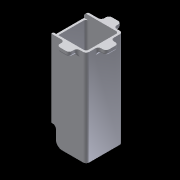
# Autodesk Inventor part: Part3
Saved by Autodesk Inventor 2012 (Build 160160000, 160)
## iProperties
Created: 2012-10-11
Part Number: Part3
Material: Default
Document SubType Name: Modeling
Designer: SONY
Density: 1 g/cm^3
Author: SONY
Autodesk Inventor part; units mm, degrees
ref_plane "YZ Plane" through (0, 0, 0) normal (1, 0, 0) x (0, 1, 0)
ref_plane "XZ Plane" through (0, 0, 0) normal (0, 1, 0) x (-1, 0, 0)
ref_plane "XY Plane" through (0, 0, 0) normal (0, 0, 1) x (1, 0, 0)
sketch "Sketch1" plane through (0, 0, 0) normal (0, 0, 1) x (1, 0, 0)
  line L0 (-50.8, 30.4821) -> (-50.8, -23.4929) projected
  arc A0 (-50.8, -23.4929) -> (-47.625, -26.6679) centre (-47.625, -23.4929) ccw projected
  line L1 (-47.625, -26.6679) -> (47.625, -26.6679) projected
  arc A1 (47.625, -26.6679) -> (50.8, -23.4929) centre (47.625, -23.4929) ccw projected
  line L2 (50.8, -23.4929) -> (50.8, 30.4821) projected
  line L3 (50.8, 30.4821) -> (25.4, 30.4821) projected
  line L4 (25.4, 30.4821) -> (25.4, 1.9071) projected
  arc A2 (22.225, -1.2679) -> (25.4, 1.9071) centre (22.225, 1.9071) ccw projected
  line L5 (22.225, -1.2679) -> (-22.225, -1.2679) projected
  arc A3 (-25.4, 1.9071) -> (-22.225, -1.2679) centre (-22.225, 1.9071) ccw projected
  line L6 (-25.4, 1.9071) -> (-25.4, 30.4821) projected
  line L7 (-25.4, 30.4821) -> (-50.8, 30.4821) projected
  arc A4 (-47.625, 87.6321) -> (-50.8, 84.4571) centre (-47.625, 84.4571) ccw projected
  line L8 (-50.8, 30.4821) -> (-50.8, 84.4571) projected
  line L9 (-25.4, 30.4821) -> (-50.8, 30.4821) projected
  line L10 (-25.4, 59.0571) -> (-25.4, 30.4821) projected
  arc A5 (-22.225, 62.2321) -> (-25.4, 59.0571) centre (-22.225, 59.0571) ccw projected
  line L11 (22.225, 62.2321) -> (-22.225, 62.2321) projected
  arc A6 (25.4, 59.0571) -> (22.225, 62.2321) centre (22.225, 59.0571) ccw projected
  line L12 (25.4, 30.4821) -> (25.4, 59.0571) projected
  line L13 (50.8, 30.4821) -> (25.4, 30.4821) projected
  line L14 (50.8, 84.4571) -> (50.8, 30.4821) projected
  arc A7 (50.8, 84.4571) -> (47.625, 87.6321) centre (47.625, 84.4571) ccw projected
  line L15 (-47.625, 87.6321) -> (47.625, 87.6321) projected
  line L16 (51.435, 0.6371) -> (24.765, 0.6371)
  line L17 (24.765, 0.6371) -> (24.765, 60.3271)
  line L18 (24.765, 60.3271) -> (51.435, 60.3271)
  line L19 (51.435, 60.3271) -> (51.435, 0.6371)
  line L20 (53.185, 0.6371) -> (23.015, 0.6371)
  line L21 (23.015, 0.6371) -> (23.015, 60.3271)
  line L22 (23.015, 60.3271) -> (53.185, 60.3271)
  line L23 (53.185, 60.3271) -> (53.185, 0.6371)
  point P0 (0, 0)
  dimension "d0" = 59.69
  dimension "d1" = 1.905
  dimension "d2" = 26.67
  dimension "d3" = 0.635
  dimension "d4" = 1.75
  dimension "d5" = 1.75
  constraints: 16 end point, 4 parallel, 2 collinear, 2 horizontal, 2 perpendicular
  measures "d0" distance of L18.end L16.start
  measures "d1" distance between parallel lines of L5 L16
  measures "d2" distance between parallel lines of L17 L19
  measures "d3" distance between parallel lines of L4 L17
  measures "d4" distance between parallel lines of L17 L21
  measures "d5" distance between parallel lines of L19 L23
extrude "Extrusion1" add sketch "Sketch1" against normal blind 26.035 contours L19 L22 L23 L20 | L20 L21 L22 L17
sketch "Sketch2" plane through (0, 0, 0) normal (0, 0, 1) x (1, 0, 0)
  line L0 (51.435, 60.3271) -> (51.435, 0.6371) projected
  line L1 (53.185, 0.6371) -> (51.435, 0.6371) projected
  line L2 (53.185, 60.3271) -> (53.185, 0.6371) projected
  line L3 (51.435, 60.3271) -> (53.185, 60.3271) projected
  line L4 (24.765, 0.6371) -> (24.765, 60.3271) projected
  line L5 (23.015, 60.3271) -> (24.765, 60.3271) projected
  line L6 (23.015, 0.6371) -> (23.015, 60.3271) projected
  line L7 (24.765, 0.6371) -> (23.015, 0.6371) projected
  point P0 (0, 0)
extrude "Extrusion2" add sketch "Sketch2" along normal blind 0.635
sketch "Sketch3" plane through (0, 0, 0.635) normal (0, 0, 1) x (1, 0, 0)
  line L0 (24.765, 0.6371) -> (23.015, 0.6371) projected
  line L1 (24.765, 60.3271) -> (24.765, 0.6371) projected
  line L2 (23.015, 60.3271) -> (24.765, 60.3271) projected
  line L3 (23.015, 0.6371) -> (23.015, 60.3271) projected
  line L4 (23.015, 60.3271) -> (53.185, 60.3271)
  line L5 (53.185, 60.3271) -> (53.185, 0.6371)
  line L6 (53.185, 0.6371) -> (23.015, 0.6371)
  line L7 (23.015, 0.6371) -> (23.015, 60.3271)
  point P0 (0, 0)
  constraints: 8 end point, 2 parallel, 1 horizontal, 1 perpendicular
extrude "Extrusion3" add sketch "Sketch3" along normal blind 1.75
sketch "Sketch4" plane through (0, 0, -26.035) normal (0, 0, -1) x (-1, 0, 0)
  line L0 (-51.435, 0.6371) -> (-51.435, 60.3271) projected
  line L1 (-53.185, 60.3271) -> (-51.435, 60.3271) projected
  line L2 (-53.185, 0.6371) -> (-53.185, 60.3271) projected
  line L3 (-51.435, 0.6371) -> (-53.185, 0.6371) projected
  line L4 (-53.185, 60.3271) -> (-23.015, 60.3271)
  line L5 (-23.015, 60.3271) -> (-23.015, 0.6371)
  line L6 (-23.015, 0.6371) -> (-53.185, 0.6371)
  line L7 (-53.185, 0.6371) -> (-53.185, 60.3271)
  point P0 (0, 0)
  constraints: 8 end point, 2 parallel, 1 horizontal, 1 perpendicular
extrude "Extrusion4" add sketch "Sketch4" along normal blind 1.75
sketch "Sketch5" plane through (0, 0, -27.785) normal (0, 0, -1) x (-1, 0, 0)
  line L0 (-53.185, 60.3271) -> (-23.015, 60.3271) projected
  line L1 (-28.3525, 60.3271) -> (-28.3525, 60.3271)
  line L2 (-23.015, 60.3271) -> (-23.015, 0.6371) projected
  line L3 (-53.185, 60.3271) -> (-23.015, 60.3271)
  line L4 (-23.015, 60.3271) -> (-23.015, 64.1371)
  line L5 (-23.015, 64.1371) -> (-53.185, 64.1371)
  line L6 (-53.185, 64.1371) -> (-53.185, 60.3271)
  point P0 (0, 0)
  dimension "d45" = 3.81
  constraints: 10 end point, 2 parallel, 2 perpendicular, 1 collinear, 1 horizontal, 1 point on line
  measures "d45" distance between parallel lines of L3 L5
extrude "Extrusion5" add sketch "Sketch5" against normal blind 1.75
sketch "Sketch6" plane through (0, 0, 2.385) normal (0, 0, 1) x (1, 0, 0)
  line L0 (51.435, 0.6371) -> (51.435, 60.3271) projected
  line L1 (53.185, 60.3271) -> (51.435, 60.3271) projected
  line L2 (24.765, 60.3271) -> (24.765, 0.6371) projected
  line L3 (51.435, 0.6371) -> (24.765, 0.6371) projected
  line L4 (53.185, 60.3271) -> (27.785, 60.3271)
  line L5 (53.185, 64.1371) -> (53.185, 60.3271) projected
  line L6 (23.015, 64.1371) -> (53.185, 64.1371) projected
  line L7 (23.015, 60.3271) -> (23.015, 64.1371) projected
  line L8 (24.765, 60.3271) -> (23.015, 60.3271) projected
  point P0 (0, 0)
  constraints: 2 end point, 1 parallel
extrude "Extrusion6" add sketch "Sketch6" against normal blind 1.75
sketch "Sketch7" plane through (53.185, 0.6371, 2.385) normal (1, 0, 0) x (0, 0, -1)
  line L0 (1.75, 63.5) -> (1.75, 59.69)
  line L1 (28.42, 59.69) -> (1.75, 59.69)
  line L2 (1.75, 59.69) -> (1.75, 63.5)
  line L3 (1.75, 63.5) -> (28.42, 63.5)
  line L4 (28.42, 63.5) -> (28.42, 59.69)
  point P0 (2.385, -0.6371)
  constraints: 10 end point, 2 parallel, 1 horizontal, 1 perpendicular
extrude "Extrusion7" add sketch "Sketch7" against normal blind 1.75
sketch "Sketch8" plane through (0, 0, -27.785) normal (0, 0, -1) x (-1, 0, 0)
  line L0 (-53.185, 0.6371) -> (-28.3525, 0.6371)
  line L1 (-28.3525, 0.6371) -> (-28.3525, -9.5229)
  line L2 (-33.4325, -14.6029) -> (-53.185, -14.6029)
  line L3 (-53.185, -14.6029) -> (-53.185, 0.6371)
  arc A0 (-33.4325, -14.6029) -> (-28.3525, -9.5229) centre (-33.4325, -9.5229) ccw
  line L4 (-23.015, 64.1371) -> (-23.015, 0.6371) projected
  point P0 (0, 0)
  dimension "d26" = 15.24
  dimension "d29" = 5.08
  dimension "d56" = 5.3375
  constraints: 8 end point, 2 parallel, 2 point on circle, 2 tangent, 1 centre point, 1 horizontal, 1 perpendicular
  measures "d26" distance between parallel lines of L0 L2
  measures "d29" radius of A0
  measures "d56" distance between parallel lines of L4 L1
extrude "Lip-1" add sketch "Sketch8" against normal blind 1.75
sketch "Sketch9" plane through (0, 0, 2.385) normal (0, 0, 1) x (1, 0, 0)
  line L0 (51.435, 0.6371) -> (51.435, 64.1371) projected
  line L1 (24.765, 60.3271) -> (24.765, 0.6371) projected
  line L2 (28.3525, 0.6371) -> (24.765, 0.6371) projected
  line L3 (28.3525, -9.5229) -> (28.3525, 0.6371) projected
  arc A0 (28.3525, -9.5229) -> (33.4325, -14.6029) centre (33.4325, -9.5229) ccw projected
  line L4 (53.185, -14.6029) -> (33.4325, -14.6029) projected
  line L5 (53.185, 0.6371) -> (53.185, -14.6029) projected
  line L6 (51.435, 0.6371) -> (53.185, 0.6371) projected
  line L7 (53.185, 0.6371) -> (28.3525, 0.6371)
  line L8 (23.015, 64.1371) -> (51.435, 64.1371) projected
  line L9 (23.015, 60.3271) -> (23.015, 64.1371) projected
  line L10 (24.765, 60.3271) -> (23.015, 60.3271) projected
  point P0 (0, 0)
  constraints: 2 end point, 1 collinear
extrude "Lip-2" add sketch "Sketch9" against normal blind 1.75 contours L6 L5 L4 A0 L3 L7
sketch "Sketch10" plane through (53.185, 0.6371, 0.635) normal (1, 0, 0) x (0, 0, -1)
  line L0 (0, 0) -> (26.67, 0)
  line L1 (26.67, 0) -> (26.67, -15.24)
  line L2 (26.67, -15.24) -> (0, -15.24)
  line L3 (0, -15.24) -> (0, 0)
  point P0 (0.635, -0.6371)
  constraints: 8 end point, 2 parallel, 1 horizontal, 1 perpendicular
extrude "Extrusion10" add sketch "Sketch10" against normal blind 1.75
fillet "Fillet1" radius 2.5 6 edges at (53.185, 24.7671, 2.385) (53.185, 24.7671, -27.785) (23.015, 64.1371, 1.51) (23.015, 64.1371, -26.91) (23.015, 32.3871, 2.385) (23.015, 32.3871, -27.785)
fillet "Fillet1" radius 2 4 edges at (51.435, 24.7671, -26.035) (51.435, 24.7671, 0.635) (24.765, 30.4821, -26.035) (24.765, 30.4821, 0.635)
sketch "Sketch11" plane through (0, 0, 2.385) normal (0, 0, 1) x (1, 0, 0)
  line L0 (53.185, -14.6029) -> (53.185, 64.1371) projected
  line L1 (35.405, 64.1371) -> (45.565, 64.1371)
  line L2 (45.565, 64.1371) -> (45.565, 60.3271)
  line L3 (45.565, 60.3271) -> (35.405, 60.3271)
  line L4 (35.405, 60.3271) -> (35.405, 64.1371)
  line L5 (50.685, 64.1371) -> (25.515, 64.1371) projected
  line L6 (19.215, 60.3271) -> (56.985, 60.3271) projected
  point P0 (0, 0)
  dimension "d36" = 10.16
  dimension "d37" = 7.62
  constraints: 8 end point, 2 collinear, 2 parallel, 1 horizontal, 1 perpendicular
  measures "d36" distance of L1.start L1.end
  measures "d37" distance between parallel lines of L0 L2
extrude "Nub1" add sketch "Sketch11" along normal blind 6.35
sketch "Sketch12" plane through (0, 0, -27.785) normal (0, 0, -1) x (-1, 0, 0)
  line L0 (-35.405, 64.1371) -> (-45.565, 64.1371) projected
  line L1 (-45.565, 60.3271) -> (-35.405, 60.3271) projected
  line L2 (-45.565, 64.1371) -> (-45.565, 60.3271) projected
  line L3 (-35.405, 60.3271) -> (-35.405, 64.1371) projected
  point P0 (0, 0)
  dimension "d47" = 10.16
  measures "d47" distance of L1.start L1.end
extrude "Nub2" add sketch "Sketch12" along normal blind 6.35
sketch "Sketch13" plane through (53.185, -14.6029, -25.285) normal (1, 0, 0) x (0, 0, -1)
  line L0 (0, 78.74) -> (-25.17, 78.74) projected
  line L1 (-25.17, 0) -> (0, 0) projected
  line L2 (-12.585, 78.74) -> (-12.585, 62.2574) construction
  line L3 (-17.665, 78.74) -> (-7.505, 78.74) construction
  line L4 (-7.505, 78.74) -> (-7.505, 74.93) construction
  line L5 (-7.505, 74.93) -> (-17.665, 74.93) construction
  line L6 (-17.665, 74.93) -> (-17.665, 78.74) construction
  line L7 (-39.1575, 72.93) -> (-39.1575, 74.93) construction
  line L8 (-39.1575, 72.93) -> (13.9875, 72.93) construction
  line L9 (13.9875, 74.93) -> (13.9875, 72.93) construction
  line L10 (-39.1575, 74.93) -> (13.9875, 74.93) construction
  line L11 (-17.665, 74.93) -> (-7.505, 74.93)
  line L12 (-7.505, 74.93) -> (-7.505, 78.74)
  line L13 (-7.505, 78.74) -> (-17.665, 78.74)
  line L14 (-17.665, 78.74) -> (-17.665, 74.93)
  point P0 (-25.285, 14.6029)
  dimension "d48" = 10.16
  dimension "d49" = 5.08
  constraints: 18 end point, 4 parallel, 3 perpendicular, 2 horizontal, 1 collinear, 1 midpoint, 1 point on line
  measures "d48" distance between parallel lines of L4 L6
  measures "d49" distance between parallel lines of L2 L6
extrude "Nub-3" add sketch "Sketch13" along normal blind 6.35
fillet "Nub-fillet" radius 2.5 12 edges at (59.535, 62.2321, -7.62) (59.535, 62.2321, -17.78) (53.185, 62.2321, -17.78) (53.185, 62.2321, -7.62) (45.565, 62.2321, 2.385) (45.565, 62.2321, 8.735) (35.405, 62.2321, 8.735) (35.405, 62.2321, 2.385) (35.405, 62.2321, -27.785) (45.565, 62.2321, -27.785) (35.405, 62.2321, -34.135) (45.565, 62.2321, -34.135)
fillet "Nub-fillet" radius 1.25 3 edges at (40.485, 60.3271, -27.785) (53.185, 60.3271, -12.7) (40.485, 60.3271, 2.385)
fillet "Nub-fllet2" radius 1.5 27 edges at (44.8328, 60.3271, -33.4028) (45.565, 60.3271, -30.96) (45.6502, 60.3271, -29.638) (46.9141, 59.8663, -28.0657) (36.1372, 60.3271, -33.4028) (35.405, 60.3271, -30.96) (35.3198, 60.3271, -29.638) (34.0559, 59.8663, -28.0657) (40.485, 60.3271, -34.135) (56.36, 60.3271, -17.78) (55.038, 60.3271, -17.8652) (53.4657, 59.8663, -19.1291) (59.535, 60.3271, -12.7) (58.8028, 60.3271, -8.3522) (56.36, 60.3271, -7.62) (55.038, 60.3271, -7.5348) (53.4657, 59.8663, -6.2709) (58.8028, 60.3271, -17.0478) (36.1372, 60.3271, 8.0028) (35.405, 60.3271, 5.56) (35.3198, 60.3271, 4.238) (34.0559, 59.8663, 2.6657) (44.8328, 60.3271, 8.0028) (45.565, 60.3271, 5.56) (45.6502, 60.3271, 4.238) (46.9141, 59.8663, 2.6657) (40.485, 60.3271, 8.735)
fillet "lip-fillet" radius 2.5 2 edges at (28.3525, 0.6371, 1.51) (28.3525, 0.6371, -26.91)
equation "\"d5\" = d4"
equation "\"d8\" = d3"
equation "\"d10\" = d5"
equation "\"d12\" = d5"
equation "\"d19\" = d4"
equation "\"d21\" = d4"
equation "\"d23\" = d4"
equation "\"d26\" = d27"
equation "\"d29\" = d28"
equation "\"d30\" = d4"
equation "\"d32\" = d4"
equation "\"d34\" = d4"
equation "\"d48\" = d47"
equation "\"d49\" = 0.5 * d47"
equation "\"d27\" = 15.24"
equation "\"d28\" = 5.08"
body "Solid1"
